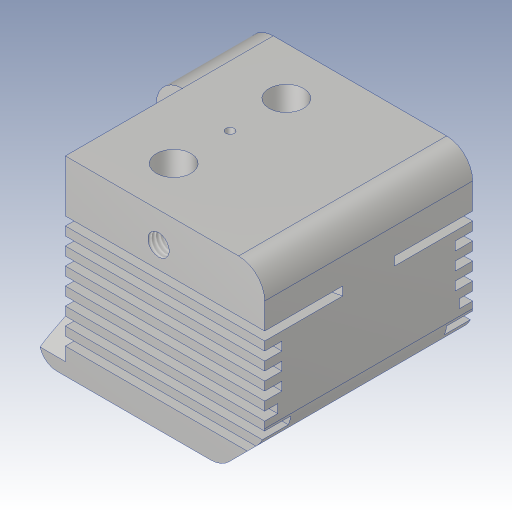
# Autodesk Inventor part: BT007_huenin20_23
Saved by Autodesk Inventor 2023.3 (Build 273359000, 359)
## iProperties
Company: HTBLA Kaindorf
RuleStatus: InUse
Created: 2023-09-14
Part Number: BT007_huenin20_23
Project: Fiberprinter-Hotend
Material: Aluminium 6061
Description: Coldend
Document SubType Name: Modeling
Designer: huenin20
Density: 2.7 g/cm^3
Appearance: Aluminium - flach
Mass: 23.9789 g
Surface Area: 65.8687 cm^2
Volume: 8.88109 cm^3
AfterDocNew0: iProperties-Editor_aufrufen
Author: nicob
Keywords: 2023
Autodesk Inventor part; units mm, degrees
ref_plane "YZ Plane" through (0, 0, 0) normal (1, 0, 0) x (0, 1, 0)
ref_plane "XZ Plane" through (0, 0, 0) normal (0, 1, 0) x (-1, 0, 0)
ref_plane "XY Plane" through (0, 0, 0) normal (0, 0, 1) x (1, 0, 0)
sketch "Skizze14" plane through (0, 0, 0) normal (1, 0, 0) x (0, 1, 0)
  line L0 (0, 0) -> (0, 22)
  line L1 (0, 22) -> (26, 22)
  line L2 (26, 0) -> (0, 0)
  line L3 (26, 0) -> (26, 22)
  line L4 (21, 0) -> (26, 5)
  dimension "d122" = 22
  dimension "d123" = 26
  dimension "d562" = 45
  dimension "d563" = 5
  constraints: 10 end point, 2 point on line, 2 vertical, 1 parallel, 1 perpendicular
  measures "d122" distance of L0.start L0.end
  measures "d123" distance of L2.start L0.start
  measures "d562" angle of L2 L4
  measures "d563" distance of L2.start L4.start
extrude "Extrusion7" add sketch "Skizze14" along normal mid plane 24 contours L0 L1 L3 L4 L2
sketch "Skizze25" plane through (-12, 0, 22) normal (0, 0, 1) x (1, 0, 0)
  line L0 (24, 0) -> (0, 0) projected
  point P0 (12, 0)
  point P1 (12, 10)
  point P2 (12, 0)
  point P3 (12, 0)
  dimension "d233" = 10
  constraints: 2 midpoint, 1 vertical alignment
  measures "d233" distance of point (12, 10) point (12, 0)
hole "Bohrung19" at (0, 10, 22) direction (0, 0, -1) diameter 1 end through all
fillet "Rundung3" radius 3 4 edges at (0, 0, 22) (0, 26, 22) (0, 26, 5) (0, 21, 0)
sketch "Skizze23" plane through (12, 0, 0) normal (0, 0, -1) x (-1, 0, 0)
  line L0 (18.5, 4) -> (5.5, 4) construction
  line L1 (5.5, 4) -> (5.5, 16) construction
  line L2 (5.5, 16) -> (18.5, 16) construction
  line L3 (18.5, 16) -> (18.5, 4) construction
  line L4 (24, 0) -> (0, 0) projected
  point P0 (12, 0)
  point P1 (12, 16)
  point P2 (18.5, 10)
  point P3 (18.5, 10)
  point P4 (5.5, 10)
  point P5 (12, 10)
  point P6 (12, 0)
  dimension "d204" = 12
  dimension "d205" = 13
  dimension "d248" = 10
  constraints: 8 end point, 5 coincident, 4 midpoint, 2 parallel, 2 vertical alignment, 1 horizontal, 1 horizontal alignment, 1 perpendicular
  measures "d204" distance of L2.end L0.start
  measures "d205" distance of L0.start L0.end
  measures "d248" distance from line of L4 point (12, 10)
hole "Bohrung16" at (6.5, 4, 0) at (6.5, 16, 0) at (-6.5, 16, 0) at (-6.5, 4, 0) direction (0, 0, 1) diameter 2.38 depth 5
sketch "Skizze24" plane through (-12, 31.5125, 22) normal (0, 0, 1) x (1, 0, 0)
  point P0 (12, -31.5125)
  point P1 (12, -21.5125)
  point P2 (5.5, -21.5125)
  point P3 (18.5, -21.5125)
  dimension "d426" = 13
  dimension "d427" = 6.5
  constraints: 2 horizontal alignment
  measures "d426" distance of point (5.5, -21.513) point (18.5, -21.513)
  measures "d427" distance of point (12, -21.513) point (18.5, -21.513)
hole "Bohrung18" at (-6.5, 10, 22) at (6.5, 10, 22) direction (0, 0, -1) diameter 2 end through all counterbore diameter 4 counterbore depth 13
sketch "Skizze28" plane through (-12, 0, 19) normal (0, -1, 0) x (1, 0, 0)
  line L0 (8, -5) -> (16, -5)
  line L1 (17, -6) -> (17, -11.1487)
  line L2 (7, -11.1487) -> (7, -6)
  line L3 (0, -19) -> (24, -19) projected
  line L4 (24, 3) -> (0, 3) projected
  arc A0 (8, -5) -> (7, -6) centre (8, -6) ccw
  arc A1 (17, -6) -> (16, -5) centre (16, -6) ccw
  line L5 (7, -11.1487) -> (7, -13.5)
  line L6 (17, -11.1487) -> (17, -13.5)
  line L7 (16, -14.5) -> (8, -14.5)
  line L8 (17, -11.25) -> (21.5, -11.25)
  line L9 (21.5, -11.25) -> (21.5, -7)
  line L10 (19.5, -5) -> (16, -5)
  line L11 (7, -11.25) -> (2.5, -11.25)
  line L12 (2.5, -11.25) -> (2.5, -7)
  line L13 (4.5, -5) -> (8, -5)
  arc A2 (4.5, -5) -> (2.5, -7) centre (4.5, -7) ccw
  arc A3 (21.5, -7) -> (19.5, -5) centre (19.5, -7) ccw
  arc A4 (16, -14.5) -> (17, -13.5) centre (16, -13.5) ccw
  arc A5 (7, -13.5) -> (8, -14.5) centre (8, -13.5) ccw
  circle A6 centre (3.8, -9.95) radius 1.5 construction
  circle A7 centre (4.5, -9.25) radius 2 construction
  arc A8 (2.5, -10.25) -> (3.5, -11.25) centre (3.5, -10.25) ccw
  arc A9 (20.5, -11.25) -> (21.5, -10.25) centre (20.5, -10.25) ccw
  circle A10 centre (15.7, -13.2) radius 1.5 construction
  circle A11 centre (8.3, -13.2) radius 1.5 construction
  circle A12 centre (9, -12.5) radius 2 construction
  circle A13 centre (15, -12.5) radius 2 construction
  point P0 (12, -19)
  point P1 (7, -5)
  point P2 (17, -5)
  point P3 (12, -19)
  point P4 (12, -19)
  point P5 (7, -14.5)
  point P6 (17, -14.5)
  point P7 (12, -5)
  point P8 (12, -19)
  point P9 (21.5, -5)
  point P10 (2.5, -5)
  point P11 (20.2, -9.95)
  dimension "d384" = 8
  dimension "d386" = 10
  dimension "d389" = 1
  dimension "d428" = 9.5
  dimension "d429" = 4.5
  dimension "d431" = 6.25
  dimension "d482" = 2
  dimension "d493" = 1.3
  dimension "d494" = 1.3
  dimension "d495" = 1.3
  dimension "d496" = 1.3
  dimension "d564" = 3
  dimension "d565" = 4
  dimension "d566" = 2
  dimension "d567" = 2
  dimension "d568" = 1.3
  dimension "d569" = 1.3
  dimension "d570" = 1.3
  dimension "d571" = 1.3
  dimension "d573" = 3
  dimension "d574" = 4
  dimension "d575" = 4
  constraints: 24 end point, 22 tangent, 18 point on line, 16 point on circle, 14 centre point, 6 perpendicular, 5 equal radius, 4 midpoint, 3 coincident, 3 horizontal, 2 horizontal alignment, 2 parallel, 1 collinear, 1 vertical, 1 vertical alignment
  measures "d384" distance between parallel lines of L4 L0
  measures "d386" distance of point (7, -5) point (17, -5)
  measures "d389" radius of A0
  measures "d428" distance between parallel lines of L0 L7
  measures "d429" distance of L8.start L8.end
  measures "d431" distance between parallel lines of L8 L0
  measures "d482" radius of A2
  measures "d493" distance from line of point (20.2, -9.95) L8
  measures "d494" distance from line of L9 point (20.2, -9.95)
  measures "d495" distance from line of L12 point (3.8, -9.95)
  measures "d496" distance from line of L11 point (3.8, -9.95)
  measures "d564" diameter of A6
  measures "d565" diameter of A7
  measures "d566" diameter of A8
  measures "d567" diameter of A9
  measures "d568" distance from line of L7 point (15.7, -13.2)
  measures "d569" distance from line of L6 point (15.7, -13.2)
  measures "d570" distance from line of L7 point (8.3, -13.2)
  measures "d571" distance from line of L5 point (8.3, -13.2)
  measures "d573" diameter of A10
  measures "d574" diameter of A12
  measures "d575" diameter of A13
extrude "Extrusion10" cut sketch "Skizze28" against normal blind 16.5 contours L0 A1 L1 L6 A4 L7 A5 L5 L2 A0 | A0 L2 L5 L11 A8 L12 A2 L13 | L10 A3 L9 A9 L8 L6 L1 A1
hole "Bohrung22" at (-8.2, 0, 9.05) at (8.2, 0, 9.05) direction (0, 1, 0) diameter 3 depth 16.5
hole "Bohrung28" at (-3.7, 0, 5.8) at (3.7, 0, 5.8) direction (0, 1, 0) diameter 3 depth 16.5
fillet "Rundung14" radius 2 1 edges at (0, 0, 0)
sketch "Skizze31" plane through (12, 0, 0) normal (1, 0, 0) x (0, 0, -1)
  arc A0 (-2, 0) -> (0, 2) centre (-2, 2) ccw projected
  line L0 (0, 2) -> (0, 19.7574) projected
  line L1 (-6.2426, 26) -> (-19, 26) projected
  line L2 (-22, 23) -> (-22, 3) projected
  arc A1 (-22, 3) -> (-19, 0) centre (-19, 3) ccw projected
  line L3 (-19, 0) -> (-2, 0) projected
  arc A2 (-19, 26) -> (-22, 23) centre (-19, 23) ccw projected
  line L4 (-0.8787, 21.8787) -> (-4.1213, 25.1213) projected
  arc A3 (0, 19.7574) -> (-0.8787, 21.8787) centre (-3, 19.7574) ccw projected
  arc A4 (-4.1213, 25.1213) -> (-6.2426, 26) centre (-6.2426, 23) ccw projected
  point P0 (0, 0)
sketch "Skizze34" plane through (12, 0, 0) normal (1, 0, 0) x (0, 0, -1)
  line L0 (-19, 0) -> (-2, 0) projected
  line L1 (-22, 23) -> (-22, 3) projected
  point P0 (0, 0)
  point P1 (-18.5, 7.25)
  point P2 (-18.5, 20.25)
  point P3 (-18.5, 13.75)
  point P4 (-22, 26)
  dimension "d484" = 3.5
  dimension "d485" = 13
  dimension "d545" = 6.5
  dimension "d560" = 13.75
  constraints: 2 vertical alignment
  measures "d484" distance from line of L1 point (-18.5, 7.25)
  measures "d485" distance of point (-18.5, 7.25) point (-18.5, 20.25)
  measures "d545" distance of point (-18.5, 20.25) point (-18.5, 13.75)
  measures "d560" distance from line of L0 point (-18.5, 13.75)
sketch "Skizze38" plane through (-12, 0, 0) normal (-1, 0, 0) x (0, 0, 1)
  point P0 (0, 0)
  point P1 (18.5, 7.25)
  point P2 (18.5, 20.25)
hole "Bohrung27" at (-12, 7.25, 18.5) at (-12, 20.25, 18.5) direction (1, 0, 0) diameter 2.459 depth 8.8 thread size "M3x0.5" class "6H" standard "ISO Metric profile"
hole "Bohrung26" at (12, 13.75, 18.5) direction (-1, 0, 0) diameter 2.459 depth 8.8 thread size "M3x0.5" class "6H" standard "ISO Metric profile"
sketch "Skizze36" plane through (-12, 0, 19) normal (0, -1, 0) x (1, 0, 0)
  line L0 (0, -17) -> (0, 0) projected
  line L1 (24, 0) -> (24, -17) projected
  line L2 (24, -3) -> (17, -3)
  line L3 (17, -3) -> (17, -4)
  line L4 (17, -4) -> (24, -4)
  line L5 (24, -5) -> (22, -5)
  line L6 (22, -5) -> (22, -6)
  line L7 (22, -6) -> (24, -6)
  line L8 (24, -7) -> (22, -7)
  line L9 (22, -7) -> (22, -8)
  line L10 (22, -8) -> (24, -8)
  line L11 (24, -9) -> (22, -9)
  line L12 (22, -9) -> (22, -10)
  line L13 (22, -10) -> (24, -10)
  line L14 (24, -13) -> (21, -13)
  line L15 (21, -13) -> (21, -14)
  line L16 (21, -14) -> (24, -14)
  line L17 (24, -11) -> (22.5, -11)
  line L18 (22.5, -11) -> (22.5, -12)
  line L19 (22.5, -12) -> (24, -12)
  line L20 (24, -15) -> (21, -15)
  line L21 (21, -15) -> (21, -16)
  line L22 (21, -16) -> (24, -16)
  point P0 (12, -19)
  point P1 (24, -13)
  point P2 (24, -9.5)
  point P3 (24, -10.5)
  point P4 (24, -8)
  point P5 (24, -7)
  point P6 (24, -5.5)
  point P7 (24, -15.5)
  point P8 (24, -14.5)
  dimension "d497" = 7
  dimension "d498" = 1
  dimension "d499" = 3
  dimension "d500" = 1
  dimension "d501" = 1
  dimension "d502" = 2
  dimension "d503" = 1
  dimension "d504" = 2
  dimension "d505" = 1
  dimension "d506" = 1
  dimension "d507" = 2
  dimension "d508" = 1
  dimension "d509" = 3
  dimension "d511" = 1
  dimension "d515" = 1
  dimension "d516" = 1.5
  dimension "d517" = 1
  dimension "d518" = 1
  dimension "d519" = 1
  dimension "d520" = 3
  dimension "d521" = 1
  constraints: 42 end point, 10 horizontal, 10 perpendicular, 13 other
  measures "d497" distance of L2.start L2.end
  measures "d498" distance of L2.end L3.end
  measures "d499" distance of point (24, 0) L2.start
  measures "d500" distance between parallel lines of L4 L5
  measures "d501" distance of L5.end L6.end
  measures "d502" distance of L5.start L5.end
  measures "d503" distance of L8.end L9.end
  measures "d504" distance of L8.start L8.end
  measures "d505" distance between parallel lines of L7 L8
  measures "d506" distance of L11.end L12.end
  measures "d507" distance of L11.start L11.end
  measures "d508" distance between parallel lines of L10 L11
  measures "d509" distance of L14.start L14.end
  measures "d511" distance of L14.end L15.end
  measures "d515" distance of L17.end L18.end
  measures "d516" distance of L17.start L17.end
  measures "d517" distance between parallel lines of L13 L17
  measures "d518" distance between parallel lines of L19 L14
  measures "d519" distance of L20.end L21.end
  measures "d520" distance of L20.start L20.end
  measures "d521" distance between parallel lines of L16 L20
extrude "Extrusion12" cut sketch "Skizze36" against normal up to surface (26 mm away)
mirror "Spiegeln1" about plane through (0, 0, 0) normal (1, 0, 0) of "Extrusion12"
chamfer "Fase7" distance 2 distance2 9 2 edges at (5, 26, 15.5) (-5, 26, 15.5) measured on face at (-4.5, 26, 15.5) measured on face at (4.5, 26, 15.5)
chamfer "Fase8" distance 2 distance2 8 6 edges at (-5, 0, 15.5) (5, 0, 15.5) (9, 0, 5.5) (9, 0, 3.5) (-9, 0, 3.5) (-9, 0, 5.5) measured on face at (-8.5, 0, 3.5) measured on face at (8.5, 0, 3.5) measured on face at (-8.5, 0, 5.5) measured on face at (4.5, 0, 15.5) measured on face at (8.5, 0, 5.5) measured on face at (-4.5, 0, 15.5)
sketch "Skizze37" plane through (-12, 0, 19) normal (0, -1, 0) x (1, 0, 0)
  line L0 (4.5, -5) -> (19.5, -5) projected
  line L1 (16, -14.5) -> (8, -14.5) projected
  circle A0 centre (12, -9.75) radius 1.5
  circle A1 centre (12, -9.75) radius 4
  line L2 (11.3008, -9.75) -> (12.6992, -9.75) construction
  line L3 (12, -9.75) -> (25, -16.3738) construction
  line L4 (25, -16.3738) -> (25, -9.75)
  line L5 (25, -9.75) -> (12, -9.75) construction
  line L6 (24.319, -17.7103) -> (25.681, -15.0373)
  line L7 (24.319, -17.7103) -> (14.623, -12.77)
  line L8 (15.9849, -10.0969) -> (25.681, -15.0373)
  line L9 (25, -8.25) -> (25, -11.25)
  line L10 (25, -11.25) -> (15.7081, -11.25)
  line L11 (15.7081, -8.25) -> (25, -8.25)
  arc A2 (16.4953, -13.724) -> (13.3397, -13.519) centre (14.6793, -17.288) ccw
  arc A3 (14.9047, -7) -> (17.8095, -8.25) centre (17.8095, -4.25) ccw
  line L12 (10.5, -6.0419) -> (10.5, 3.9581)
  line L13 (10.5, 3.9581) -> (13.5, 3.9581)
  line L14 (13.5, 3.9581) -> (13.5, -6.0419)
  line L15 (25, -8.25) -> (25, -7.25)
  line L16 (25, -7.25) -> (15.1225, -7.25)
  line L17 (13.5, 3.9581) -> (25, 3.9581)
  line L18 (25, 3.9581) -> (25, -7.25)
  point P0 (12, -19)
  point P1 (12, -5)
  point P2 (12, 3.9581)
  point P3 (10.5, -5)
  point P4 (13.5, -5)
  point P5 (15.1637, -7.25)
  dimension "d531" = 8
  dimension "d528" = 9.5
  dimension "d529" = 4.75
  dimension "d530" = 3
  dimension "d533" = 27
  dimension "d534" = 13
  dimension "d535" = 3
  dimension "d536" = 3
  dimension "d537" = 4
  dimension "d538" = 4
  dimension "d541" = 27
  dimension "d542" = 3
  dimension "d543" = 10
  dimension "d544" = 1
  constraints: 34 end point, 10 perpendicular, 5 midpoint, 4 point on circle, 3 centre point, 3 coincident, 2 horizontal, 2 point on line, 2 tangent, 2 vertical, 2 vertical alignment, 1 parallel, 13 other
  measures "d528" distance between parallel lines of L0 L1
  measures "d529" distance from line of L0 point (12, -9.75)
  measures "d530" diameter of A0
  measures "d533" angle of L5 L3
  measures "d534" distance from line of L4 A0.centre
  measures "d535" distance of L6.start L6.end
  measures "d536" distance of L9.start L9.end
  measures "d537" radius of A2
  measures "d538" radius of A3
  measures "d541" angle of L2 L7
  measures "d542" distance of L12.end L13.end
  measures "d543" distance of L13.end L14.end
  measures "d544" distance of L9.start L15.end
extrude "Extrusion13" cut sketch "Skizze37" against normal blind 3 contours L12 L13 L14 L0 | L14 L17 L18 L16 A3 A1 | A1 L7 A2 | A3 L16 A1 | A1 L10 L8 L4 L6 L7 | L15 L11 A3 L16 | L16 A3 L11 A1 | A1 L8 L10 | L9 L4 L10 L8 A1 L11 | L10 L4 L8
